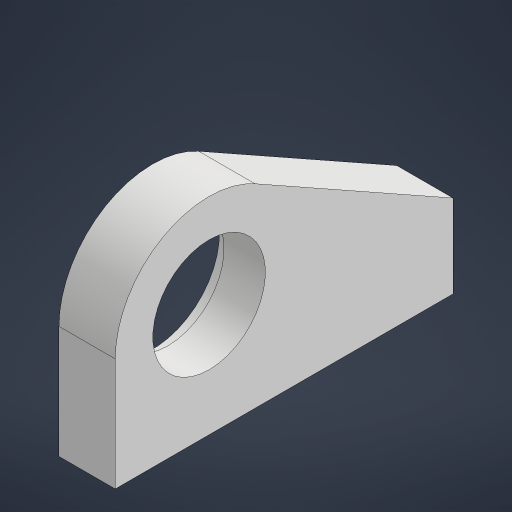
# Autodesk Inventor part: Stand
Saved by Autodesk Inventor 2024.2 (Build 282272000, 272)
## iProperties
Created: 2024-01-12
Part Number: Stand
Material: 一般
Document SubType Name: Modeling
Designer: Hanaoka
Density: 1 g/cm^3
Appearance: 既定
Author: Hanaoka
Autodesk Inventor part; units mm, degrees
ref_plane "YZ Plane" through (0, 0, 0) normal (1, 0, 0) x (0, 1, 0)
ref_plane "XZ Plane" through (0, 0, 0) normal (0, 1, 0) x (-1, 0, 0)
ref_plane "XY Plane" through (0, 0, 0) normal (0, 0, 1) x (1, 0, 0)
sketch "スケッチ1" plane through (0, 0, 0) normal (1, 0, 0) x (0, 1, 0)
  circle A0 centre (0, 0) radius 3.55
  arc A1 (4.3581, -2.4508) -> (0, 5) centre (0, 0) ccw
  line L0 (4.3581, -2.4508) -> (-1.5743, -13)
  line L1 (-1.5743, -13) -> (-6, -13)
  line L2 (-6, -13) -> (-6, 5)
  line L3 (-6, 5) -> (0, 5)
  circle A2 centre (0, 0) radius 3
  dimension "d0" = 7.1
  dimension "d1" = 5
  dimension "d2" = 18
  dimension "d3" = 6
  dimension "d6" = 6
  constraints: 8 end point, 3 centre point, 3 coincident, 3 point on circle, 2 horizontal, 2 tangent, 1 vertical
  measures "d0" diameter of A0
  measures "d1" radius of A1
  measures "d2" distance of L1.end L2.end
  measures "d3" distance from line of L2 point (0, 0)
  measures "d6" diameter of A2
extrude "押し出し1" add sketch "スケッチ1" along normal blind 3 contours A0 | L0 L1 L2 L3 A1
extrude "押し出し2" cut sketch "スケッチ1" along normal blind 0.8 contours A0 | A2
